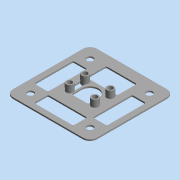
# Autodesk Inventor part: SensorMount_top
Saved by Autodesk Inventor 2015 (Build 190159000, 159)
## iProperties
Created: 2015-08-15
Part Number: SensorMount_top
Material: Generic
Document SubType Name: Modeling
Designer: Raphael
Appearance: Generic
Author: Raphael
Autodesk Inventor part; units mm, degrees
ref_plane "YZ Plane" through (0, 0, 0) normal (1, 0, 0) x (0, 1, 0)
ref_plane "XZ Plane" through (0, 0, 0) normal (0, 1, 0) x (-1, 0, 0)
ref_plane "XY Plane" through (0, 0, 0) normal (0, 0, 1) x (1, 0, 0)
sketch "Sketch1" plane through (0, 0, 0) normal (0, 1, 0) x (-1, 0, 0)
  line L0 (0, 0) -> (60, 0)
  line L1 (60, 0) -> (60, -60)
  line L2 (60, -60) -> (0, -60)
  line L3 (0, -60) -> (0, 0)
  circle A0 centre (51.2132, -8.7868) radius 2.25
  circle A1 centre (8.7868, -51.2132) radius 2.25
  circle A2 centre (8.7868, -8.7868) radius 2.25
  circle A3 centre (51.2132, -51.2132) radius 2.25
  line L4 (51.2132, -8.7868) -> (8.7868, -51.2132) construction
  line L5 (51.2132, -51.2132) -> (8.7868, -8.7868) construction
  line L6 (51.2132, -8.7868) -> (8.7868, -8.7868) construction
  line L7 (21, -24.5) -> (39, -24.5) construction
  line L8 (39, -24.5) -> (39, -35.5) construction
  line L9 (39, -35.5) -> (21, -35.5) construction
  line L10 (21, -35.5) -> (21, -24.5) construction
  line L11 (30, 0) -> (30, -60) construction
  circle A4 centre (21, -24.5) radius 1.75
  circle A5 centre (21, -35.5) radius 1.75
  line L12 (19, -22.5) -> (41, -22.5) construction
  line L13 (41, -22.5) -> (41, -52.5) construction
  line L14 (41, -52.5) -> (19, -52.5) construction
  line L15 (19, -52.5) -> (19, -22.5) construction
  line L16 (21, -24.5) -> (19, -24.5) construction
  line L17 (21, -24.5) -> (21, -22.5) construction
  line L18 (39, -24.5) -> (41, -24.5) construction
  circle A6 centre (39, -24.5) radius 1.75
  circle A7 centre (39, -35.5) radius 1.75
  arc A8 (24, -30) -> (36, -30) centre (30, -30) ccw
  line L19 (19, -52.5) -> (41, -52.5)
  line L20 (41, -52.5) -> (41, -38.5196)
  line L21 (41, -38.5196) -> (19, -38.5196)
  line L22 (19, -38.5196) -> (19, -52.5)
  circle A9 centre (21, -24.5) radius 2.5
  circle A10 centre (21, -35.5) radius 2.5
  circle A11 centre (39, -24.5) radius 2.5
  circle A12 centre (39, -35.5) radius 2.5
  line L23 (24, -30) -> (36, -30) construction
  line L24 (36, -30) -> (36, -22.75)
  line L25 (36, -22.75) -> (24, -22.75)
  line L26 (24, -22.75) -> (24, -30)
  line L27 (40.75, -26.2854) -> (40.75, -33.7146)
  line L28 (37.25, -33.7146) -> (37.25, -26.2854)
  line L29 (4, -16) -> (14, -16)
  line L30 (14, -16) -> (14, -44)
  line L31 (14, -44) -> (4, -44)
  line L32 (4, -44) -> (4, -16)
  line L33 (16, -4) -> (44, -4)
  line L34 (44, -4) -> (44, -14)
  line L35 (44, -14) -> (16, -14)
  line L36 (16, -14) -> (16, -4)
  line L37 (56, -16) -> (46, -16)
  line L38 (46, -16) -> (46, -44)
  line L39 (46, -44) -> (56, -44)
  line L40 (56, -44) -> (56, -16)
  point P0 (60, -30)
  point P1 (39, -30)
  point P2 (30, -24.5)
  dimension "d0" = 4.5
  dimension "d1" = 4.5
  dimension "d2" = 4.5
  dimension "d3" = 4.5
  dimension "d4" = 60
  dimension "d5" = 60
  dimension "d6" = 18
  dimension "d7" = 11
  dimension "d8" = 60
  dimension "d9" = 3.5
  dimension "d10" = 3.5
  dimension "d11" = 22
  dimension "d12" = 30
  dimension "d13" = 3.5
  dimension "d14" = 3.5
  dimension "d15" = 12
  dimension "d16" = 5
  dimension "d17" = 5
  dimension "d18" = 5
  dimension "d19" = 5
  dimension "d26" = 4
  dimension "d27" = 10
  dimension "d28" = 16
  dimension "d29" = 16
  dimension "d30" = 4
  dimension "d31" = 16
  dimension "d32" = 16
  dimension "d33" = 10
  constraints: 82 end point, 15 parallel, 13 centre point, 12 perpendicular, 10 coincident, 7 horizontal, 7 midpoint, 6 point on circle, 6 tangent, 5 point on line, 4 symmetric about line, 3 equal length, 2 horizontal alignment, 1 vertical, 1 vertical alignment
  measures "d0" diameter of A0
  measures "d1" diameter of A1
  measures "d2" diameter of A2
  measures "d3" diameter of A3
  measures "d4" distance of L4.end L4.start
  measures "d5" distance of L5.end L5.start
  measures "d6" distance of L8.end L9.end
  measures "d7" distance of L7.end L8.end
  measures "d8" distance of L0.end L1.end
  measures "d9" diameter of A4
  measures "d10" diameter of A5
  measures "d11" distance of L13.end L14.end
  measures "d12" distance of L12.end L13.end
  measures "d13" diameter of A6
  measures "d14" diameter of A7
  measures "d15" diameter of A8
  measures "d16" diameter of A9
  measures "d17" diameter of A10
  measures "d18" diameter of A11
  measures "d19" diameter of A12
  measures "d26" distance between parallel lines of L32 L3
  measures "d27" distance of L30.end L31.end
  measures "d28" distance between parallel lines of L29 L0
  measures "d29" distance between parallel lines of L2 L31
  measures "d30" distance between parallel lines of L33 L0
  measures "d31" distance between parallel lines of L34 L1
  measures "d32" distance between parallel lines of L36 L3
  measures "d33" distance between parallel lines of L33 L35
extrude "Extrusion1" add sketch "Sketch1" along normal blind 1 contours L0 L1 L2 L3
extrude "Extrusion2" add sketch "Sketch1" along normal blind 6 contours A9 | A10 | A11 | A12
fillet "Fillet1" radius 1 18 edges at (-41, 0.5, -52.5) (-41, 0.5, -38.5196) (-19, 0.5, -38.5196) (-19, 0.5, -52.5) (-36, 0.5, -22.75) (-24, 0.5, -22.75) (-44, 0.5, -4) (-44, 0.5, -14) (-56, 0.5, -44) (-56, 0.5, -16) (-46, 0.5, -44) (-46, 0.5, -16) (-16, 0.5, -4) (-16, 0.5, -14) (-4, 0.5, -44) (-4, 0.5, -16) (-14, 0.5, -16) (-14, 0.5, -44)
fillet "Fillet2" radius 5 4 edges at (0, 0.5, -60) (-60, 0.5, -60) (-60, 0.5, 0) (0, 0.5, 0)
body "Solid1"
